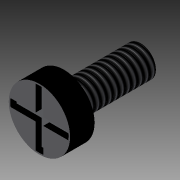
# Autodesk Inventor part: M2x6_D963
Saved by Autodesk Inventor 2015 (Build 190159000, 159)
## iProperties
Created: 2015-01-10
Part Number: M2x6_D963
Material: Generic
Document SubType Name: Modeling
Designer: ice
Density: 1 g/cm^3
Appearance: Default
Mass: 0.0343986 g
Surface Area: 0.826843 cm^2
Volume: 0.0343986 cm^3
Author: ice
Autodesk Inventor part; units mm, degrees
ref_plane "YZ Plane" through (0, 0, 0) normal (1, 0, 0) x (0, 1, 0)
ref_plane "XZ Plane" through (0, 0, 0) normal (0, 1, 0) x (-1, 0, 0)
ref_plane "XY Plane" through (0, 0, 0) normal (0, 0, 1) x (1, 0, 0)
ref_plane "Work Plane4" through (0, 0, 0) normal (0, -1, 0) x (1, 0, 0)
sketch "Sketch2" plane through (0, 0, 0) normal (0, -1, 0) x (1, 0, 0)
  circle A0 centre (0, 0) radius 2
  dimension "d23" = 4
  constraints: 1 centre point
  measures "d23" diameter of A0
extrude "Extrusion4" add sketch "Sketch2" against normal blind 1.6
ref_plane "Work Plane2" through (0, 0, 0) normal (0, -1, 0) x (1, 0, 0)
sketch "Sketch4" plane through (0, 0, 0) normal (0, -1, 0) x (1, 0, 0)
  arc A0 (-0.25, -1.8835) -> (0.25, -1.8835) centre (0, 0) ccw
  arc A1 (0.25, 1.8835) -> (-0.25, 1.8835) centre (0, 0) ccw
  line L0 (0.25, 0.25) -> (1.8835, 0.25)
  line L1 (-0.25, 0.25) -> (-1.8835, 0.25)
  arc A2 (-0.25, -1.8835) -> (0.25, -1.8835) centre (0, 0) ccw
  arc A3 (1.8835, -0.25) -> (1.8835, 0.25) centre (0, 0) ccw
  arc A4 (0.25, 1.8835) -> (-0.25, 1.8835) centre (0, 0) ccw
  arc A5 (-1.8835, 0.25) -> (-1.8835, -0.25) centre (0, 0) ccw
  line L2 (1.8835, -0.25) -> (0.25, -0.25)
  line L3 (-0.25, -0.25) -> (-1.8835, -0.25)
  line L4 (-0.25, -1.8835) -> (-0.25, -0.25)
  line L5 (-0.25, 0.25) -> (-0.25, 1.8835)
  line L6 (0.25, -1.8835) -> (0.25, -0.25)
  line L7 (0.25, 0.25) -> (0.25, 1.8835)
  constraints: 16 end point, 12 point on circle, 6 centre point, 2 coincident, 1 horizontal
extrude "Extrusion5" cut sketch "Sketch4" against normal blind 0.4
ref_plane "Work Plane5" through (0, 1.6, 0) normal (0, 1, 0) x (1, 0, 0)
sketch "Sketch5" plane through (0, 1.6, 0) normal (0, 1, 0) x (1, 0, 0)
  circle A0 centre (0, 0) radius 1
  dimension "d24" = 2
  constraints: 1 centre point, 1 coincident
  measures "d24" diameter of A0
extrude "Extrusion6" add sketch "Sketch5" along normal blind 5
ref_plane "Work Plane6" through (0, 1.6, 0) normal (0, 1, 0) x (1, 0, 0)
thread "Thread3" size "M2x0.4" class "6g" standard "ANSI Metric M Profile" full length
body "Solid2"
